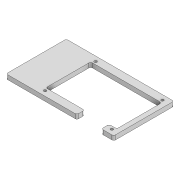
# Autodesk Inventor part: Top PMMA
Saved by Autodesk Inventor 2020 (Build 240168000, 168)
## iProperties
Created: 2021-07-01
Part Number: Top PMMA
Material: Generic
Document SubType Name: Modeling
Designer: ferrerx
Density: 1 g/cm^3
Appearance: Default
Author: ferrerx
Autodesk Inventor part; units mm, degrees
ref_plane "YZ Plane" through (0, 0, 0) normal (1, 0, 0) x (0, 1, 0)
ref_plane "XZ Plane" through (0, 0, 0) normal (0, 1, 0) x (-1, 0, 0)
ref_plane "XY Plane" through (0, 0, 0) normal (0, 0, 1) x (1, 0, 0)
sketch "Sketch1" plane through (0, 0, 0) normal (0, 1, 0) x (-1, 0, 0)
  line L0 (-2.27, 0) -> (120.44, 0)
  line L1 (120.44, 0) -> (120.44, -68.57)
  line L2 (120.44, -68.57) -> (-2.27, -68.57)
  line L3 (-2.27, -68.57) -> (-2.27, 0)
  line L4 (120.44, -66.57) -> (120.44, -2)
  line L5 (0, -68.57) -> (118.44, -68.57)
  line L6 (-2.27, -2.27) -> (-2.27, -66.3)
  circle A0 centre (81.55, -63.09) radius 1.5
  circle A1 centre (81.55, -63.09) radius 1.5
  line L7 (70.44, -68.57) -> (15.73, -68.57)
  line L8 (51, 0) -> (75, 0)
  line L9 (26, 0) -> (51, 0)
  line L10 (84, -60) -> (79, -60)
  line L11 (79, -60) -> (79, -8.7337)
  line L12 (79, -8.7337) -> (84, -8.7337)
  line L13 (84, -8.7337) -> (84, -60)
  line L14 (8, -60) -> (3, -60)
  line L15 (3, -60) -> (3, -8.7337)
  line L16 (3, -8.7337) -> (8, -8.7337)
  line L17 (8, -8.7337) -> (8, -60)
  circle A2 centre (5.25, -63.09) radius 1.5
  circle A3 centre (5.35, -5.47) radius 1.5
  circle A4 centre (81.55, -5.47) radius 1.5
  circle A5 centre (81.55, -5.47) radius 1.5
  circle A6 centre (5.35, -5.47) radius 1.5
  circle A7 centre (5.25, -63.09) radius 1.5
  dimension "d20" = 3
  dimension "d27" = 3
  dimension "d28" = 3
  dimension "d29" = 3
  dimension "d30" = 68.57
  constraints: 36 end point, 8 centre point, 6 parallel, 4 collinear, 4 concentric, 4 horizontal, 3 perpendicular, 3 point on line
  measures "d20" diameter of A0
  measures "d27" diameter of A2
  measures "d28" diameter of A3
  measures "d29" diameter of A4
  measures "d30" distance of L0.end L1.end
extrude "Extrusion1" add sketch "Sketch1" along normal blind 5
fillet "Fillet4" radius 2 4 edges at (-120.44, 2.5, -68.57) (-120.44, 2.5, 0) (2.27, 2.5, -68.57) (2.27, 2.5, 0)
sketch "Sketch7" plane through (0, 5, 0) normal (0, 1, 0) x (1, 0, 0)
  line L0 (-117.44, 63.57) -> (-87.44, 63.57)
  line L1 (-87.44, 63.57) -> (-87.44, 5)
  line L2 (-87.44, 5) -> (-117.44, 5)
  line L3 (-117.44, 5) -> (-117.44, 63.57)
  line L4 (-120.44, 66.57) -> (-120.44, 2) projected
  line L5 (0.27, 68.57) -> (-118.44, 68.57) projected
  line L6 (-118.44, 0) -> (0.27, 0) projected
  point P0 (0, 0)
  dimension "d67" = 30
  dimension "d68" = 3
  dimension "d69" = 5
  dimension "d70" = 5
  constraints: 8 end point, 2 parallel, 1 horizontal, 1 perpendicular
  measures "d67" distance of L1.end L2.end
  measures "d68" distance between parallel lines of L4 L3
  measures "d69" distance between parallel lines of L5 L0
  measures "d70" distance between parallel lines of L6 L2
extrude "Extrusion6" [suppressed]
fillet "Fillet8" [suppressed]
sketch "Sketch8" plane through (0, 5, 0) normal (0, 1, 0) x (1, 0, 0)
  line L0 (-79, 60) -> (-8, 60)
  line L1 (-8, 60) -> (-8, 8.7337)
  line L2 (-8, 8.7337) -> (-79, 8.7337)
  line L3 (-79, 8.7337) -> (-79, 60)
  line L4 (-8, 8.7337) -> (-8, 60) projected
  line L5 (0.27, 68.57) -> (-118.44, 68.57) projected
  line L6 (-79, 60) -> (-79, 8.7337) projected
  line L7 (-3, 8.7337) -> (-8, 8.7337) projected
  line L8 (-8, 60) -> (-3, 60) projected
  point P0 (0, 0)
  constraints: 8 end point, 4 collinear, 2 parallel, 1 horizontal, 1 perpendicular
extrude "Extrusion7" cut sketch "Sketch8" against normal blind 10
sketch "Sketch9" plane through (0, 5, 0) normal (0, 1, 0) x (1, 0, 0)
  line L0 (-3, 8.7337) -> (-84, 8.7337) projected
  line L1 (-118.44, 0) -> (0.27, 0) projected
  line L2 (-39.73, 8.7337) -> (-11.73, 8.7337)
  line L3 (-11.73, 8.7337) -> (-11.73, 0)
  line L4 (-11.73, 0) -> (-39.73, 0)
  line L5 (-39.73, 0) -> (-39.73, 8.7337)
  line L6 (2.27, 2) -> (2.27, 66.57) projected
  point P0 (0, 0)
  point P1 (-79, 8.57)
  point P2 (-8, 8.57)
  point P3 (-39.73, 0)
  point P4 (-11.73, 8.57)
  point P5 (-11.73, 8.7337)
  point P6 (-79, 8.871)
  point P7 (-8, 8.871)
  point P8 (-11.73, 8.871)
  point P9 (-11.73, 8.7337)
  dimension "d78" = 28
  dimension "d81" = 14
  dimension "d82" = 8.7338
  constraints: 8 end point, 2 parallel, 1 horizontal, 1 perpendicular, 1 point on line, 2 other
  measures "d78" distance between parallel lines of L5 L3
  measures "d81" distance between parallel lines of L6 L3
  measures "d82" distance of L4.end L2.start
extrude "Extrusion8" cut sketch "Sketch9" against normal blind 5
fillet "Fillet9" radius 2 8 edges at (-84, 2.5, -60) (-3, 2.5, -60) (-3, 2.5, -8.7337) (-11.73, 2.5, -8.7337) (-11.73, 2.5, 0) (-39.73, 2.5, -8.7337) (-39.73, 2.5, 0) (-84, 2.5, -8.7337)
body "Solid1"
